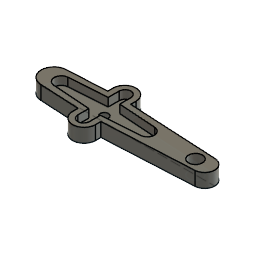
base_brazo_servo (Autodesk Fusion 360 design; units mm, degrees)
part number: 2026-03-17-23-48-58-358
Autodesk Fusion 360 part; units mm, degrees
sketch "Boceto1" plane through (0, 0, 0) normal (0, 1, 0) x (1, 0, 0)
  line L0 (0, 0) -> (0, 17.5982) construction
  line L1 (0, 0) -> (24, 0) construction
  line L2 (0, 0) -> (0, 7.35) construction
  line L3 (-4.15, -5.3969) -> (-18.2868, -4.6482)
  arc A0 (-18.2868, 4.6482) -> (-18.2868, -4.6482) centre (-18.2, 0) ccw
  line L4 (-4.15, 5.3969) -> (-18.2868, 4.6482)
  line L5 (-4.15, 7.35) -> (-4.15, 5.3969)
  arc A1 (4.15, 7.35) -> (-4.15, 7.35) centre (0, 7.35) ccw
  line L6 (4.15, 5.3969) -> (4.15, 7.35)
  line L7 (4.15, 5.3969) -> (36.5066, 3.6833)
  line L8 (4.15, -5.3969) -> (36.5066, -3.6833)
  line L9 (4.15, -5.3969) -> (4.15, -7.35)
  arc A2 (-4.15, -7.35) -> (4.15, -7.35) centre (0, -7.35) ccw
  line L10 (-4.15, -7.35) -> (-4.15, -5.3969)
  line L11 (40, 9) -> (40, -14)
  arc A3 (18.2443, -4.6505) -> (18.6472, -4.6291) centre (18.2, 0) ccw
  arc A4 (18.6472, 4.6291) -> (18.2443, 4.6505) centre (18.2, 0) ccw
  arc A5 (36.5066, -3.6833) -> (36.5066, 3.6833) centre (36.3115, 0) ccw
  arc A6 (2.1, 7.5) -> (-2.1, 7.5) centre (0, 7.5) ccw
  arc A7 (-2.1, -7.5) -> (2.1, -7.5) centre (0, -7.5) ccw
  line L12 (0, -7.5) -> (0, 7.5) construction
  line L13 (2.1, 3.4965) -> (15.7278, 2.5438)
  line L14 (2.1, -3.4965) -> (15.7278, -2.5438)
  line L15 (2.1, -7.5) -> (2.1, -3.4965)
  line L16 (2.1, 3.4965) -> (2.1, 7.5)
  arc A8 (15.7278, -2.5438) -> (15.7278, 2.5438) centre (15.55, 0) ccw
  line L17 (-2.1, 3.4965) -> (-15.7278, 2.5438)
  line L18 (-2.1, -3.4965) -> (-15.7278, -2.5438)
  arc A9 (-15.7278, 2.5438) -> (-15.7278, -2.5438) centre (-15.55, 0) ccw
  line L19 (-2.1, 7.5) -> (-2.1, 3.4965)
  line L20 (-2.1, -3.4965) -> (-2.1, -7.5)
  line L21 (-3.5359, 3.4965) -> (-2.1, 3.4965) construction
  point P0 (0, 9.5)
  point P1 (0, -9.5)
  point P2 (-20.85, 0)
  point P3 (20.85, 0)
  point P4 (0, 9.6)
  point P5 (0, -9.6)
  point P6 (0, 11.5)
  point P7 (-18.1, 0)
  point P8 (18.1, 0)
  dimension "d10" = 40
  dimension "d26" = 4.2
  dimension "d32" = 5.1
  dimension "d33" = 18.1
  dimension "d35" = 9.6
  constraint vertical L0
  constraint coincident L0.start L1.start
  constraint perpendicular L0 L1
  constraint coincident L0 L2.end
  constraint perpendicular L1 L2
  constraint vertical L11
  constraint tangent A1 L6
  constraint tangent L5 A1
  constraint tangent L9 A2
  constraint tangent A2 L10
  constraint coincident A4.end L7
  constraint coincident A3.start L8
  constraint tangent L7 A5
  constraint tangent L11 A5
  constraint tangent L8 A5
  constraint coincident L8 A3.end
  constraint concentric A3 A4
  constraint coincident L7 A4.start
  constraint tangent A6 L16
  constraint tangent A6 L19
  constraint parallel L16 L19
  constraint tangent A7 L20
  constraint tangent A7 L15
  constraint coincident L2 A6.centre
  constraint perpendicular L1 L12
  constraint midpoint L12 L0.start
  constraint midpoint A6 P4
  constraint midpoint A7 P5
  constraint midpoint A1 P6
  constraint coincident L1 A8.centre
  constraint tangent L13 A8
  constraint symmetric L1 L13.start L14.start
  constraint symmetric L1 L13.end L14.end
  constraint collinear L15 L16
  constraint symmetric L12 L13.start L17.start
  constraint symmetric L12 L13.end L17.end
  constraint symmetric L12 L14.start L18.start
  constraint symmetric L12 L14.end L18.end
  constraint symmetric L12 A8 A9
  constraint collinear L19 L20
  constraint midpoint A9 P7
  constraint midpoint A8 P8
  measures "d10" distance of L0.start L11
  measures "d26" distance of L16 L19
  measures "d32" diameter of A8
  measures "d33" distance of L0.start P8
  measures "d35" distance of L0.start P4
extrude "Extruir1" add sketch "Boceto1" along normal blind 5 contours L3 A0 L4 L5 A1 L6 L7 L8 L9 A2 L10 A5
sketch "Boceto2" plane through (0, 0, 0) normal (0, -1, 0) x (1, 0, 0)
  line L0 (36.5066, 3.6833) -> (4.15, 5.3969)
  line L1 (4.15, 5.3969) -> (4.15, 7.35)
  arc A0 (4.15, 7.35) -> (-4.15, 7.35) centre (0, 7.35) ccw
  line L2 (-4.15, 7.35) -> (-4.15, 5.3969)
  line L3 (-4.15, 5.3969) -> (-18.2868, 4.6482)
  arc A1 (-18.2868, 4.6482) -> (-18.2868, -4.6482) centre (-18.2, 0) ccw
  line L4 (-18.2868, -4.6482) -> (-4.15, -5.3969)
  line L5 (-4.15, -5.3969) -> (-4.15, -7.35)
  arc A2 (-4.15, -7.35) -> (4.15, -7.35) centre (0, -7.35) ccw
  line L6 (4.15, -7.35) -> (4.15, -5.3969)
  line L7 (4.15, -5.3969) -> (36.5066, -3.6833)
  arc A3 (36.5066, -3.6833) -> (36.5066, 3.6833) centre (36.3115, 0) ccw
  line L8 (4.15, 5.3969) -> (36.5066, 3.6833)
  line L9 (0, 0) -> (48.5, 0) construction
  circle A4 centre (33, 0) radius 2.5
  arc A5 (2.1, 7.5) -> (-2.1, 7.5) centre (0, 7.5) ccw
  arc A6 (-2.1, -7.5) -> (2.1, -7.5) centre (0, -7.5) ccw
  line L10 (2.1, -3.4965) -> (2.1, -7.5)
  line L11 (-2.1, -7.5) -> (-2.1, -3.4965)
  line L12 (-2.1, -3.4965) -> (-15.7278, -2.5438)
  arc A7 (-15.7278, 2.5438) -> (-15.7278, -2.5438) centre (-15.55, 0) ccw
  line L13 (-15.7278, 2.5438) -> (-2.1, 3.4965)
  line L14 (-2.1, 3.4965) -> (-2.1, 7.5)
  line L15 (2.1, 7.5) -> (2.1, 3.4965)
  line L16 (2.1, 3.4965) -> (15.7278, 2.5438)
  arc A8 (15.7278, -2.5438) -> (15.7278, 2.5438) centre (15.55, 0) ccw
  line L17 (15.7278, -2.5438) -> (2.1, -3.4965)
  point P0 (34.0022, 2.75)
  point P1 (32.9604, 2.4997)
  dimension "d21" = 5
  dimension "d22" = 33
  constraint coincident L9.start origin
  constraint horizontal L9
  constraint coincident L9 A4.centre
  constraint coincident A4 P1
  measures "d21" diameter of A4
  measures "d22" distance of L9.start A4.centre
extrude "Extruir3" cut sketch "Boceto2" against normal through all contours A4
extrude "Extrude4" add sketch "Boceto2" against normal blind 2 contours A5 A6 L10 L11 L12 A7 L13 L14 L15 L16 A8 L17
sketch "Boceto3" plane through (0, 2, 0) normal (0, 1, 0) x (-1, 0, 0)
  arc A0 (2.1, 7.5) -> (-2.1, 7.5) centre (0, 7.5) ccw
  line L0 (-2.1, 7.5) -> (-2.1, 3.4965)
  line L1 (-2.1, 3.4965) -> (-15.7278, 2.5438)
  arc A1 (-15.7278, 2.5438) -> (-15.7278, -2.5438) centre (-15.55, 0) ccw
  line L2 (-15.7278, -2.5438) -> (-2.1, -3.4965)
  line L3 (-2.1, -3.4965) -> (-2.1, -7.5)
  arc A2 (-2.1, -7.5) -> (2.1, -7.5) centre (0, -7.5) ccw
  line L4 (2.1, -7.5) -> (2.1, -3.4965)
  line L5 (2.1, -3.4965) -> (15.7278, -2.5438)
  arc A3 (15.7278, -2.5438) -> (15.7278, 2.5438) centre (15.55, 0) ccw
  line L6 (15.7278, 2.5438) -> (2.1, 3.4965)
  line L7 (2.1, 3.4965) -> (2.1, 7.5)
  circle A4 centre (0, 0) radius 1.5
  dimension "d38" = 3
  constraint coincident A4.centre origin
  measures "d38" diameter of A4
extrude "Extruir5" cut sketch "Boceto3" against normal through all contours A4
sketch "Boceto4" plane through (0, 0, 0) normal (0, -1, 0) x (1, 0, 0)
  circle A0 centre (0, 0) radius 1.5
  circle A1 centre (33, 0) radius 2.5
  line L0 (36.5066, 3.6833) -> (4.15, 5.3969)
  line L1 (4.15, 5.3969) -> (4.15, 7.35)
  arc A2 (4.15, 7.35) -> (-4.15, 7.35) centre (0, 7.35) ccw
  line L2 (-4.15, 7.35) -> (-4.15, 5.3969)
  line L3 (-4.15, 5.3969) -> (-18.2868, 4.6482)
  arc A3 (-18.2868, 4.6482) -> (-18.2868, -4.6482) centre (-18.2, 0) ccw
  line L4 (-18.2868, -4.6482) -> (-4.15, -5.3969)
  line L5 (-4.15, -5.3969) -> (-4.15, -7.35)
  arc A4 (-4.15, -7.35) -> (4.15, -7.35) centre (0, -7.35) ccw
  line L6 (4.15, -7.35) -> (4.15, -5.3969)
  line L7 (4.15, -5.3969) -> (36.5066, -3.6833)
  arc A5 (36.5066, -3.6833) -> (36.5066, 3.6833) centre (36.3115, 0) ccw
  line L8 (-22.849, 0) -> (40, 0) construction
  constraint midpoint A3 L8.start
  constraint midpoint A5 L8.end
equation "d35 = ( 19.2 / 2 ) * 1 mm"
